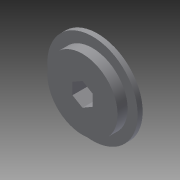
# Autodesk Inventor part: Tube End Cap
Saved by Autodesk Inventor 2014 (Build 180170000, 170)
## iProperties
Created: 2014-01-07
Part Number: Tube End Cap
Material: Generic
Document SubType Name: Modeling
Designer: Andrew Toennies
Density: 1 g/cm^3
Appearance: Default
Author: Andrew Toennies
Autodesk Inventor part; units mm, degrees
ref_plane "YZ Plane" through (0, 0, 0) normal (1, 0, 0) x (0, 1, 0)
ref_plane "XZ Plane" through (0, 0, 0) normal (0, 1, 0) x (-1, 0, 0)
ref_plane "XY Plane" through (0, 0, 0) normal (0, 0, 1) x (1, 0, 0)
sketch "Sketch1" plane through (0, 0, 0) normal (0, 0, 1) x (1, 0, 0)
  circle A0 centre (0, 0) radius 28.575
  line L0 (0, 7.3323) -> (6.35, 3.6662)
  line L1 (6.35, 3.6662) -> (6.35, -3.6662)
  line L2 (6.35, -3.6662) -> (0, -7.3323)
  line L3 (0, -7.3323) -> (-6.35, -3.6662)
  line L4 (-6.35, -3.6662) -> (-6.35, 3.6662)
  line L5 (-6.35, 3.6662) -> (0, 7.3323)
  dimension "d0" = 57.15
  dimension "d1" = 12.7
  constraints: 12 end point, 2 coincident, 1 centre point, 1 vertical, 13 other
  measures "d0" diameter of A0
  measures "d1" distance between parallel lines of L1 L4
extrude "Extrusion1" add sketch "Sketch1" along normal blind 3.175
sketch "Sketch3" plane through (0, 0, 3.175) normal (0, 0, 1) x (1, 0, 0)
  line L0 (6.35, 3.6662) -> (6.35, -3.6662) projected
  line L1 (6.35, -3.6662) -> (0, -7.3323) projected
  line L2 (0, -7.3323) -> (-6.35, -3.6662) projected
  line L3 (-6.35, -3.6662) -> (-6.35, 3.6662) projected
  line L4 (-6.35, 3.6662) -> (0, 7.3323) projected
  line L5 (0, 7.3323) -> (6.35, 3.6662) projected
  circle A0 centre (0, 0) radius 28.575 projected
  circle A1 centre (0, 0) radius 22.225
  dimension "d8" = 44.45
  constraints: 1 centre point, 1 coincident
  measures "d8" diameter of A1
extrude "Extrusion3" add sketch "Sketch3" along normal blind 6.35 contours A1
body "Solid1"
